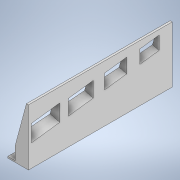
# Autodesk Inventor part: SortBoard-Frame
Saved by Autodesk Inventor 2020 (Build 240168000, 168)
## iProperties
Created: 2020-03-07
Part Number: SortBoard-Frame
Material: Типовые
Document SubType Name: Modeling
Designer: CSS38
Density: 1 g/cm^3
Appearance: По умолчанию
Author: CSS38
Autodesk Inventor part; units mm, degrees
ref_plane "YZ Plane" through (0, 0, 0) normal (1, 0, 0) x (0, 1, 0)
ref_plane "XZ Plane" through (0, 0, 0) normal (0, 1, 0) x (-1, 0, 0)
sketch "Эскиз1" plane through (0, 0, 0) normal (0, 1, 0) x (-1, 0, 0)
  line L0 (8.75, 95.5) -> (-8.75, 95.5)
  line L1 (-8.75, 95.5) -> (-8.75, -95.5)
  line L2 (-8.75, -95.5) -> (8.75, -95.5)
  line L3 (8.75, -95.5) -> (8.75, 95.5)
  line L4 (8.75, -95.5) -> (-8.75, 95.5) construction
  line L5 (-8.75, -95.5) -> (8.75, 95.5) construction
  point P0 (0, 0)
  point P1 (0, 0)
  dimension "d0" = 17.5
  dimension "d1" = 191
  constraints: 12 end point, 2 parallel, 1 coincident, 1 horizontal, 1 midpoint, 1 perpendicular
  measures "d0" distance of L1.end L2.end
  measures "d1" distance of L2.end L0.start
extrude "Выдавливание1" add sketch "Эскиз1" along normal blind 75
sketch "Эскиз2" plane through (-8.75, 0, -95.5) normal (-1, 0, 0) x (0, 0, 1)
  line L0 (191, 0) -> (191, 75) construction
  line L1 (191, 20) -> (0, 20)
  line L2 (0, 0) -> (0, 75) construction
  line L3 (0, 0) -> (191, 0) construction
  point P0 (95.5, 0)
  dimension "d4" = 20
  constraints: 2 end point, 2 point on line, 1 horizontal
  measures "d4" distance between parallel lines of L3 L1
ref_plane "РабПлоскость1" through (-8.75, 20, 95.5) normal (-0.9659258, 0.258819, 0) x (0, 0, -1)
split "Разделение1" plane through (-8.75, 20, 95.5) removes the side toward (-0.9659258, 0.258819, 0)
sketch "Эскиз3" plane through (5.9872, 75, -95.5) normal (-0.9659258, 0.258819, 0) x (0, 0, 1)
  line L0 (0, -56.9402) -> (0, 0) construction
  line L1 (0, 0) -> (191, 0) construction
  line L2 (191, 0) -> (191, -56.9402) construction
  line L3 (191, -56.9402) -> (0, -56.9402) construction
  line L4 (191, -71.7294) -> (191, 0.7151) construction
  line L5 (191, -53.9402) -> (0, -30.4883) construction
  line L6 (0, -71.7294) -> (0, 0.7151) construction
  line L7 (17.5, -22.562) -> (43, -25.693)
  line L8 (43, -25.693) -> (43, -8.5653)
  line L9 (43, -8.5653) -> (17.5, -5.4343)
  line L10 (17.5, -5.4343) -> (17.5, -22.562)
  line L11 (47, 0) -> (47, -56.9402) construction
  line L12 (191, -56.9402) -> (0, -56.9402) construction
  line L13 (94, 0) -> (94, -56.9402) construction
  line L14 (142, 0) -> (142, -56.9402) construction
  line L15 (43, -8.5653) -> (47, -8.5653) construction
  line L16 (60.5, -27.8417) -> (60.5, -9.2028)
  line L17 (60.5, -9.2028) -> (90, -12.8249)
  line L18 (90, -12.8249) -> (90, -31.4639)
  line L19 (90, -31.4639) -> (60.5, -27.8417)
  line L20 (90, -12.8249) -> (94, -12.8249) construction
  line L21 (105, -33.3056) -> (105, -13.6592)
  line L22 (105, -13.6592) -> (138, -17.7111)
  line L23 (138, -17.7111) -> (138, -37.3575)
  line L24 (138, -37.3575) -> (105, -33.3056)
  line L25 (138, -17.7111) -> (142, -17.7111) construction
  line L26 (149.5, -17.1081) -> (149.5, -38.7695)
  line L27 (149.5, -38.7695) -> (187, -43.374)
  line L28 (187, -43.374) -> (187, -21.7125)
  line L29 (187, -21.7125) -> (149.5, -17.1081)
  line L30 (187, -21.7125) -> (191, -21.7125) construction
  point P0 (95.5, -73.994)
  dimension "d6" = 3
  dimension "d7" = 7
  dimension "d8" = 10
  dimension "d9" = 25.5
  dimension "d10" = 27
  dimension "d11" = 4
  dimension "d12" = 29.5
  dimension "d13" = 28.5
  dimension "d14" = 33
  dimension "d15" = 29.5
  dimension "d16" = 37.5
  dimension "d17" = 31.5
  dimension "d36" = 49
  dimension "d37" = 48
  dimension "d38" = 47
  constraints: 48 end point, 13 parallel, 9 point on line, 5 perpendicular, 4 vertical, 3 collinear, 3 horizontal alignment, 1 horizontal
  measures "d6" distance of L2.end L5.start
  measures "d7" angle of L3 L5
  measures "d8" distance between parallel lines of L5 L7
  measures "d9" distance between parallel lines of L8 L10
  measures "d10" distance between parallel lines of L5 L9
  measures "d11" distance of L8.end L15.end
  measures "d12" distance between parallel lines of L18 L16
  measures "d13" distance between parallel lines of L5 L17
  measures "d14" distance between parallel lines of L21 L23
  measures "d15" distance between parallel lines of L5 L22
  measures "d16" horizontal distance of L26.end L27.end
  measures "d17" distance between parallel lines of L5 L29
  measures "d36" distance between parallel lines of L14 L2
  measures "d37" distance between parallel lines of L13 L14
  measures "d38" distance between parallel lines of L11 L13
extrude "Выдавливание2" cut sketch "Эскиз3" against normal through all
sketch "Эскиз5" plane through (0, 0, 0) normal (0, 1, 0) x (-1, 0, 0)
  line L0 (8.75, -95.5) -> (-8.75, -95.5) construction
  line L1 (-8.75, -95.5) -> (-8.75, 95.5) construction
  line L2 (-8.75, 95.5) -> (8.75, 95.5) construction
  line L3 (8.75, 95.5) -> (8.75, -95.5) projected
  line L4 (8.75, -95.5) -> (18.75, -95.5)
  line L5 (18.75, -95.5) -> (18.75, 85.5)
  line L6 (18.75, 95.5) -> (8.75, 95.5)
  line L7 (8.75, 95.5) -> (8.75, -95.5) construction
  line L8 (18.75, 85.5) -> (18.75, 95.5)
  line L9 (24.25, 0) -> (-14.25, 0) construction
  point P0 (0, 0)
  point P1 (8.75, 95.5)
  dimension "d26" = 10
  constraints: 10 end point, 3 parallel, 3 perpendicular, 1 collinear, 1 horizontal
  measures "d26" distance of L6.start L6.end
extrude "Выдавливание5" add sketch "Эскиз5" along normal blind 2
sketch "Эскиз4" plane through (5.9872, 75, -95.5) normal (-0.9659258, 0.258819, 0) x (0, 0, 1)
  line L0 (191, 0.7151) -> (0, 0.7151) construction
  line L1 (95.5, 0.7151) -> (95.5, -56.9402) construction
  line L2 (191, -56.9402) -> (0, -56.9402) construction
  line L3 (191, -71.7294) -> (191, 0.7151) construction
  line L4 (0, -71.7294) -> (0, 0.7151) construction
  line L5 (191, -28.1126) -> (0, -28.1126) construction
  line L6 (191, -76.2587) -> (191, -56.9402) construction
  circle A0 centre (5, -51.9402) radius 0.5
  circle A1 centre (5, -4.2849) radius 0.5
  line L7 (0, -56.9402) -> (0, 0) projected
  line L8 (0, -56.9402) -> (10, -56.9402)
  line L9 (10, -56.9402) -> (10, -46.9402)
  line L10 (10, -46.9402) -> (0, -46.9402)
  line L11 (0, -46.9402) -> (0, -56.9402)
  line L12 (10, -56.9402) -> (0, -46.9402) construction
  line L13 (0, -56.9402) -> (10, -46.9402) construction
  circle A2 centre (186, -4.2849) radius 0.5
  point P0 (95.5, -73.994)
  point P1 (95.5, -28.1126)
  dimension "d46" = 10
  dimension "d47" = 1
  constraints: 16 end point, 6 midpoint, 4 perpendicular, 3 centre point, 2 parallel, 2 point on line, 2 symmetric about line, 1 coincident, 1 horizontal, 2 other
  measures "d46" distance of L10.end L9.end
  measures "d47" diameter of A0
hole "Отверстие1" at (-7.4559, 24.8296, -90.5) at (4.8782, 70.8611, -90.5) at (4.8782, 70.8611, 90.5) direction (0.9659258, -0.258819, 0) diameter 1 depth 2.5 tip angle 118 countersink diameter 1.5 countersink angle 90
sketch "Эскиз6" plane through (0, 2, 0) normal (0, 1, 0) x (1, 0, 0)
  line L0 (-8.75, -95.5) -> (-8.75, 95.5) construction
  line L1 (-18.75, 95.5) -> (-8.75, 95.5) construction
  line L2 (-18.75, -95.5) -> (-18.75, 95.5) construction
  line L3 (-8.75, -95.5) -> (-18.75, -95.5) construction
  line L4 (8.75, -95.5) -> (-8.75, -95.5) construction
  line L5 (8.75, 95.5) -> (8.75, -95.5) construction
  line L6 (-8.75, 95.5) -> (8.75, 95.5) construction
  line L7 (-8.75, -95.5) -> (-18.75, -95.5) construction
  line L8 (-18.75, -95.5) -> (-18.75, -85.5) construction
  line L9 (-18.75, -85.5) -> (-8.75, -85.5) construction
  line L10 (-8.75, -85.5) -> (-8.75, -95.5) construction
  circle A0 centre (-13.75, -85.5) radius 0.5
  circle A1 centre (-13.75, -36.5) radius 0.5
  circle A2 centre (-13.75, 11.5) radius 0.5
  circle A3 centre (-13.75, 58.5) radius 0.5
  point P0 (0, 0)
  dimension "d50" = 1
  dimension "d51" = 49
  dimension "d52" = 48
  dimension "d53" = 47
  constraints: 8 end point, 4 centre point, 3 equal radius, 3 vertical alignment, 2 parallel, 2 perpendicular, 1 collinear, 1 horizontal, 1 midpoint
  measures "d50" diameter of A0
  measures "d51" distance of A1.centre A0.centre
  measures "d52" distance of A2.centre A1.centre
  measures "d53" distance of A3.centre A2.centre
hole "Отверстие2" at (-13.75, 2, -58.5) at (-13.75, 2, -11.5) at (-13.75, 2, 36.5) at (-13.75, 2, 85.5) direction (0, -1, 0) diameter 1 end through all countersink diameter 1.5 countersink angle 90
